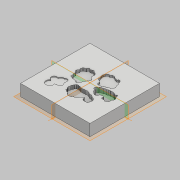
# Autodesk Inventor part: Placa - Pitting 8, 6, 4 mm
Saved by Autodesk Inventor 2017 (Build 210142000, 142)
## iProperties
Part Number: Placa - Pitting 8, 6, 4 mm
Material: Genérico
Document SubType Name: Modeling
Designer: franc
Density: 1 g/cm^3
Appearance: Valor por defecto
Author: franc
Autodesk Inventor part; units mm, degrees
sketch "Boceto1" plane through (0, 0, 0) normal (0, 0, 1) x (1, 0, 0)
  line L0 (-75, 75) -> (75, 75)
  line L1 (75, 75) -> (75, -75)
  line L2 (75, -75) -> (-75, -75)
  line L3 (-75, -75) -> (-75, 75)
  line L4 (-75, 75) -> (75, -75) construction
  line L5 (75, 75) -> (-75, -75) construction
  point P0 (0, 0)
  dimension "d0" = 150
  dimension "d1" = 150
  constraints: 12 end point, 2 midpoint, 2 parallel, 1 horizontal, 1 perpendicular
  measures "d0" distance of L1.end L2.end
  measures "d1" distance of L0.end L1.end
extrude "Extrusión1" add sketch "Boceto1" along normal blind 25
sketch "Boceto2" plane through (0, 0, 25) normal (0, 0, 1) x (1, 0, 0)
  arc A0 (-11.0344, -4.1529) -> (-7.3863, 2.1356) centre (-18.0668, 4.1292) ccw
  arc A1 (-16.961, 25.1242) -> (-22.9607, 25.8965) centre (-20.0106, 25.1242) ccw
  circle A2 centre (-7.3442, -35.1165) radius 6.2507
  circle A3 centre (13.9685, -26.75) radius 8.4379
  circle A4 centre (-5.4904, -28.3974) radius 10.2647
  circle A5 centre (28.1956, -31.2499) radius 7.5216
  line L0 (-10.3669, 20.5412) -> (-10.3669, 19.2268)
  arc A6 (-7.3863, 2.1356) -> (-6.9655, 10.156) centre (-8.2443, 6.2019) ccw
  arc A7 (-22.3012, 27.1373) -> (-23.6491, 26.0767) centre (-22.2011, 25.6233) ccw
  arc A8 (-19.3358, -10.2298) -> (-14.5163, -11.5352) centre (-16.8883, -10.7431) ccw
  line L1 (-19.3358, -10.2298) -> (-24.6054, -10.2298)
  line L2 (-36.2262, 0.8834) -> (-34.5458, -1.3804)
  line L3 (-34.5458, -1.3804) -> (-34.5458, -7.1252)
  line L4 (14.8502, 6.7404) -> (18.0606, 6.4094)
  line L5 (18.0606, 6.4094) -> (19.4279, 7.262)
  line L6 (19.4279, 7.262) -> (20.2199, 9.0168)
  line L7 (23.6015, 9.8645) -> (25.5289, 10.5419)
  line L8 (25.5289, 10.5419) -> (26.5856, 11.7252)
  line L9 (31.2983, 12.5697) -> (29.4701, 12.2785)
  line L10 (-16.1702, -25.1039) -> (-16.3929, -23.0404)
  line L11 (-16.3929, -23.0404) -> (-14.7648, -22.1301)
  line L12 (-14.7648, -22.1301) -> (-14.9554, -20.3645)
  line L13 (-14.9554, -20.3645) -> (-14.2662, -19.407)
  line L14 (-14.2662, -19.407) -> (-13.8943, -19.1991)
  line L15 (-13.8943, -19.1991) -> (-12.6342, -17.1397)
  line L16 (-12.6342, -17.1397) -> (-11.5457, -16.7312)
  line L17 (-11.5457, -16.7312) -> (-11.0269, -16.3628)
  line L18 (-11.0269, -16.3628) -> (-8.6609, -15.6485)
  line L19 (-8.6609, -15.6485) -> (-8.1522, -16.3649)
  line L20 (-8.1522, -16.3649) -> (-7.179, -16.9604)
  line L21 (-7.179, -16.9604) -> (-6.3627, -16.7139)
  line L22 (-6.3627, -16.7139) -> (-5.2537, -17.1518)
  line L23 (-5.2537, -17.1518) -> (-3.661, -16.9799)
  line L24 (-3.661, -16.9799) -> (-2.8768, -17.4597)
  line L25 (-2.8768, -17.4597) -> (-2.5669, -17.4263)
  line L26 (-2.5669, -17.4263) -> (-1.8791, -18.0701)
  line L27 (-1.8791, -18.0701) -> (-0.4363, -17.9144)
  arc A9 (14.9645, -18.3711) -> (6.4882, -22.8455) centre (11.3882, -21.862) ccw
  line L28 (21.6742, -34.9977) -> (21.8468, -36.5964)
  line L29 (21.8468, -36.5964) -> (23.261, -38.5813)
  line L30 (23.261, -38.5813) -> (24.8469, -38.9543)
  line L31 (24.8469, -38.9543) -> (26.9941, -39.761)
  line L32 (26.9941, -39.761) -> (29.4478, -39.0938)
  line L33 (31.0761, -39.4342) -> (32.2812, -38.95)
  line L34 (32.2812, -38.95) -> (33.894, -38.3019)
  line L35 (33.894, -38.3019) -> (34.3786, -35.5328)
  line L36 (-15.91, -32.7799) -> (-14.2339, -35.1404)
  line L37 (-14.2339, -35.1404) -> (-14.6894, -37.5049)
  line L38 (-2.9514, -45.6744) -> (-1.568, -46.6254)
  line L39 (-1.568, -46.6254) -> (0.1168, -45.9937)
  line L40 (0.1168, -45.9937) -> (2.6364, -46.3842)
  line L41 (2.6364, -46.3842) -> (4.6941, -45.1115)
  line L42 (4.6941, -45.1115) -> (4.9123, -43.7036)
  line L43 (4.9123, -43.7036) -> (6.8933, -42.9228)
  line L44 (6.8933, -42.9228) -> (10.0465, -42.8161)
  line L45 (10.0465, -42.8161) -> (13.1551, -40.2162)
  line L46 (13.1551, -40.2162) -> (14.0738, -39.071)
  line L47 (-10.7259, 14.3072) -> (-10.3669, 19.2268)
  line L48 (-10.7259, 14.3072) -> (-6.9655, 10.156)
  arc A10 (-26.1502, 25.8478) -> (-31.0641, 23.7116) centre (-28.6459, 24.8689) ccw
  line L49 (-24.6054, -10.2298) -> (-24.993, -9.6424)
  arc A11 (-35.539, 4.8505) -> (-35.692, 4.3492) centre (-33.8779, 4.0695) ccw
  line L50 (-36.2262, 0.8834) -> (-35.692, 4.3492)
  arc A12 (-30.4493, -7.8763) -> (-27.711, -9.5469) centre (-28.6753, -8.0479) ccw
  line L51 (-27.711, -9.5469) -> (-24.993, -9.6424)
  line L52 (-14.5163, -11.5352) -> (-12.1601, -9.4017)
  line L53 (-12.1601, -9.4017) -> (-11.2518, -6.9841)
  line L54 (-11.2518, -6.9841) -> (-11.0344, -4.1529)
  arc A13 (6.6761, 36.3198) -> (-0.2794, 32.8296) centre (4.074, 32.8296) ccw
  arc A14 (22.905, 34.8382) -> (18.5308, 35.7568) centre (20.1427, 32.5585) ccw
  arc A15 (8.6973, 8.2933) -> (12.2264, 6.0827) centre (11.3139, 8.5482) ccw
  arc A16 (32.9522, 15.0287) -> (33.5355, 22.8391) centre (31.2983, 19.0792) ccw
  line L55 (18.6123, 35.6981) -> (13.427, 39.4304)
  line L56 (13.427, 39.4304) -> (8.6849, 39.0584)
  line L57 (8.6849, 39.0584) -> (6.6761, 36.3198)
  arc A17 (31.2983, 30.4273) -> (30.4083, 31.9042) centre (28.5434, 29.7736) ccw
  arc A18 (30.4083, 31.9042) -> (30.0875, 33.8638) centre (28.5434, 32.605) ccw
  line L58 (31.2983, 12.5697) -> (32.9522, 15.0287)
  line L59 (33.5355, 22.8391) -> (32.9522, 27.7606)
  line L60 (32.9522, 27.7606) -> (31.2983, 30.4273)
  line L61 (22.905, 34.8382) -> (24.6909, 37.4935)
  line L62 (24.6909, 37.4935) -> (26.7637, 37.7391)
  line L63 (26.7637, 37.7391) -> (28.6342, 36.4811)
  line L64 (28.6342, 36.4811) -> (30.0875, 33.8638)
  arc A19 (0.7523, 20.9449) -> (2.8506, 15.7654) centre (3.4789, 19.0347) ccw
  line L65 (0.7523, 20.9449) -> (-0.6025, 22.7946)
  line L66 (-0.6025, 22.7946) -> (-1.0615, 25.5005)
  line L67 (-1.0615, 25.5005) -> (-1.7041, 26.3777)
  line L68 (-1.7041, 26.3777) -> (-1.9392, 28.7752)
  line L69 (-1.9392, 28.7752) -> (-1.3828, 31.426)
  line L70 (-1.3828, 31.426) -> (-0.2794, 32.8296)
  line L71 (26.5856, 11.7252) -> (29.4701, 12.2785)
  line L72 (20.2199, 9.0168) -> (23.6015, 9.8645)
  line L73 (14.8502, 6.7404) -> (12.2264, 6.0827)
  line L74 (8.6973, 8.2933) -> (8.2165, 11.7264)
  line L75 (8.2165, 11.7264) -> (7.4399, 13.916)
  line L76 (7.4399, 13.916) -> (6.3098, 15.0287)
  line L77 (6.3098, 15.0287) -> (3.9341, 15.373)
  line L78 (3.9341, 15.373) -> (2.8341, 15.7714)
  line L79 (31.0761, -39.4342) -> (29.4478, -39.0938)
  circle A20 centre (3.3523, -20.9379) radius 3.0912
  line L80 (-0.4363, -17.9144) -> (1.7212, -18.3121)
  line L81 (7.7472, -18.4385) -> (6.221, -17.0658)
  line L82 (6.221, -17.0658) -> (3.9955, -17.9144)
  line L83 (-16.1702, -25.1039) -> (-17.2089, -28.1905)
  line L84 (-17.2089, -28.1905) -> (-16.6895, -31.1511)
  line L85 (-16.6895, -31.1511) -> (-15.91, -32.7799)
  line L86 (14.0738, -39.071) -> (16.2036, -34.8865)
  line L87 (-2.9514, -45.6744) -> (-5.4704, -43.9429)
  line L88 (-5.4704, -43.9429) -> (-7.3249, -41.3672)
  line L89 (-14.6894, -37.5049) -> (-11.4344, -39.8433)
  circle A21 centre (22.4012, -26.4541) radius 6.0506
  arc A22 (22.0049, -13.4452) -> (31.9159, -11.1821) centre (26.7121, -11.2264) ccw
  arc A23 (42.1714, 7.9866) -> (36.5075, 7.6109) centre (39.669, 2.8307) ccw
  arc A24 (40.8851, -11.6301) -> (43.6251, -15.8739) centre (42.4114, -13.6511) ccw
  arc A25 (16.4775, 0.9995) -> (18.2031, -6.3978) centre (16.4775, -2.9004) ccw
  arc A26 (28.8098, 5.9272) -> (24.0602, 5.1714) centre (26.8077, 3.2069) ccw
  line L90 (16.4775, 0.9995) -> (17.7722, 3.6109)
  line L91 (17.7722, 3.6109) -> (24.0602, 5.1714)
  line L92 (28.8098, 5.9272) -> (32.412, 7.6109)
  line L93 (32.412, 7.6109) -> (35.4398, 8.3623)
  line L94 (35.4398, 8.3623) -> (36.5075, 7.6109)
  line L95 (18.2031, -6.3978) -> (17.9323, -11.1184)
  line L96 (17.9323, -11.1184) -> (22.0049, -13.4452)
  line L97 (31.9159, -11.1821) -> (35.344, -9.5798)
  line L98 (35.344, -9.5798) -> (38.3277, -9.7509)
  line L99 (38.3277, -9.7509) -> (40.5132, -10.8344)
  line L100 (40.5132, -10.8344) -> (40.8851, -11.6301)
  line L101 (-34.5458, -7.1252) -> (-30.4493, -7.8763)
  line L102 (-28.6459, 24.8689) -> (-31.8894, 23.3166)
  line L103 (-35.6203, 22.3199) -> (-36.8319, 20.9513)
  line L104 (-36.8319, 20.9513) -> (-38.2729, 18.0026)
  line L105 (-38.2729, 18.0026) -> (-37.0565, 13.916)
  line L106 (-20.0106, 25.1242) -> (-24.7992, 26.3777)
  line L107 (-24.7992, 26.3777) -> (-28.6459, 24.8689)
  line L108 (-20.0106, 25.1242) -> (-15.5788, 25.1242)
  line L109 (-15.5788, 25.1242) -> (-11.706, 23.6863)
  line L110 (-11.706, 23.6863) -> (-10.3669, 20.5412)
  line L111 (-37.0565, 13.916) -> (-39.3642, 10.71)
  line L112 (-39.3642, 10.71) -> (-39.6889, 7.9866)
  line L113 (-39.6889, 7.9866) -> (-38.4131, 6.2019)
  line L114 (-38.4131, 6.2019) -> (-35.539, 4.8505)
  line L115 (-31.8894, 23.3166) -> (-35.6203, 22.3199)
  arc A27 (55.0414, -7.8763) -> (55.0414, 0.7691) centre (52.3726, -3.5536) ccw
  line L116 (55.0414, -7.8763) -> (55.0414, -13.9716)
  line L117 (55.0414, -13.9716) -> (52.3726, -15.8739)
  line L118 (52.3726, -15.8739) -> (48.8143, -17.6112)
  line L119 (48.8143, -17.6112) -> (46.2694, -15.8739)
  line L120 (46.2694, -15.8739) -> (43.6251, -15.8739)
  line L121 (53.7676, 3.6163) -> (55.0414, 0.7691)
  line L122 (53.7676, 3.6163) -> (53.3652, 7.0942)
  line L123 (53.3652, 7.0942) -> (51.1107, 7.0942)
  line L124 (51.1107, 7.0942) -> (48.2495, 4.7401)
  line L125 (48.2495, 4.7401) -> (44.3379, 7.9866)
  line L126 (44.3379, 7.9866) -> (42.1714, 7.9866)
  circle A28 centre (-36.976, -29.9119) radius 9.0778
  circle A29 centre (-39.051, -24.0292) radius 6.1257
  circle A30 centre (-33.4509, -21.5465) radius 5.428
  circle A31 centre (-31.0641, -33.6727) radius 5.148
  circle A32 centre (-44.7477, -42.1665) radius 8.0415
  circle A33 centre (-48.1478, -29.3292) radius 6.1623
  point P0 (17.0707, 20.1326)
  point P1 (-18.3224, 22.5846)
  point P2 (32.6375, -25.18)
  constraints: 254 end point, 60 point on circle, 32 centre point, 18 point on line, 11 parallel, 10 perpendicular, 3 horizontal, 2 tangent, 1 coincident, 1 vertical, 6 other
extrude "Extrusión6" cut sketch "Boceto2" against normal blind 8 contours A2 A4 | L89 L37 L36 L85 L84 L83 L10 L11 L12 L13 L14 L15 L16 L17 L18 L19 L20 L21 L22 L23 L24 L25 L26 L27 L80 A20 A4 A2 | A2 A4 A20 A9 A3 L86 L46 L45 L44 L43 L42 L41 L40 L39 L38 L87 L88 | A4 A20 A2 | A2 A4 | A20 A4 | A4 A20 | A20 L82 L81 A9 | A9 A3 | A3 A21 | A21 A5 A3 | A3 A5 A21 | A3 A5 A21 | A5 A21 A3 | A3 A5 | A5 A21 | A5 L35 L34 L33 L79 L32 L31 L30 L29 L28
extrude "Extrusión7" cut sketch "Boceto2" against normal blind 6 contours L54 L53 L52 A8 L1 L49 L51 A12 L101 L3 L2 L50 A11 L114 L113 L112 L111 L105 L104 L103 L115 L102 L107 L106 L108 L109 L110 L0 L47 L48 A6 A0 | L108 L106 A1 | A1 L106 A7 | L107 L102 A10
extrude "Extrusión8" cut sketch "Boceto2" against normal blind 4 contours L73 A15 L74 L75 L76 L77 L78 A19 L65 L66 L67 L68 L69 L70 A13 L57 L56 L55 A14 L61 L62 L63 L64 A18 A17 L60 L59 A16 L58 L9 L71 L8 L7 L72 L6 L5 L4
extrude "Extrusión9" cut sketch "Boceto2" against normal blind 10 contours L96 L95 A25 L90 L91 A26 L92 L93 L94 A23 L126 L125 L124 L123 L122 L121 A27 L116 L117 L118 L119 L120 A24 L100 L99 L98 L97 A22
extrude "Extrusión10" cut sketch "Boceto2" against normal blind 2 contours A28 A31 | A28 A31 | A31 A28 A32 A33 A29 A30 | A30 A29 A28 | A28 A29 A30 | A32 A33 A28 | A28 A33 A32 | A29 A30 A28 | A28 A30 A29 | A29 A33 A28 A30 | A33 A32 A28 | A28 A32 A33 | A32 A28 A29 A33 | A28 A33 A29 A30 | A29 A28 A33 | A32 A33 A29 A28 | A28 A29 A33
